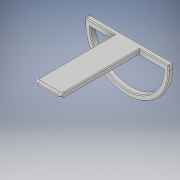
# Autodesk Inventor part: band_stand
Saved by Autodesk Inventor 2019 (Build 230136000, 136)
## iProperties
Created: 2020-03-30
Part Number: band_stand
Material: Generic
Document SubType Name: Modeling
Designer: tdeith
Density: 1 g/cm^3
Appearance: Default
Author: tdeith
Autodesk Inventor part; units mm, degrees
ref_plane "YZ Plane" through (0, 0, 0) normal (1, 0, 0) x (0, 1, 0)
ref_plane "XZ Plane" through (0, 0, 0) normal (0, 1, 0) x (-1, 0, 0)
ref_plane "XY Plane" through (0, 0, 0) normal (0, 0, 1) x (1, 0, 0)
sketch "Sketch1" plane through (0, 0, 0) normal (0, 0, 1) x (0, 1, 0)
  line L0 (0, 15) -> (0, -15)
  line L1 (0, -15) -> (6, -15)
  line L2 (6, -15) -> (6, 15)
  line L3 (6, 15) -> (0, 15)
  line L4 (5, 50) -> (0, 50)
  line L5 (0, 50) -> (0, -50)
  line L6 (0, -50) -> (5, -50)
  line L7 (6, -49) -> (6, 49)
  line L8 (-61.2414, 0) -> (17.4485, 0) projected
  arc A0 (0, 50) -> (0, -50) centre (0, 0) ccw
  arc A1 (0, 44) -> (0, -44) centre (0, 0) ccw
  arc A2 (6, 49) -> (5, 50) centre (5, 49) ccw
  arc A3 (5, -50) -> (6, -49) centre (5, -49) ccw
  dimension "d0" = 30
  dimension "d1" = 6
  dimension "d4" = 100
  dimension "d5" = 6
  dimension "d6" = 1
  constraints: 16 end point, 8 point on circle, 4 centre point, 4 tangent, 3 coincident, 2 collinear, 2 point on line, 1 equal radius, 1 horizontal, 1 midpoint, 1 parallel, 1 vertical, 1 other
  measures "d0" distance between parallel lines of L3 L1
  measures "d1" distance between parallel lines of L2 L0
  measures "d4" distance between parallel lines of L6 L4
  measures "d5" radial gap between concentric circles of A0 A1
  measures "d6" radius of A2
extrude "Extrusion1" add sketch "Sketch1" along normal blind 100 contours L3 L2 L8 L0 | L8 L2 L1 L0
extrude "Extrusion2" add sketch "Sketch1" along normal blind 6 contours L5 L4 A2 L7 L3 | A1 L8 A0 L5 | L1 L7 A3 L6 L5 | A1 L5 A0 L8
fillet "Fillet1" radius 2 4 edges at (0, 0, 100) (15, 3, 100) (0, 6, 100) (-15, 3, 100)
fillet "Fillet1" radius 1 19 edges at (-15, 0, 53) (-15, 6, 53) (0, 6, 0) (15, 6, 53) (15, 0, 53) (0, 0, 0) (-49.7071, 5.7071, 0) (-50, 2.5, 0) (0, -50, 0) (50, 2.5, 0) (49.7071, 5.7071, 0) (0, -50, 6) (0, -44, 6) (-50, 2.5, 6) (-49.7071, 5.7071, 6) (49.7071, 5.7071, 6) (50, 2.5, 6) (32, 6, 6) (-32, 6, 6)
body "Solid1"
